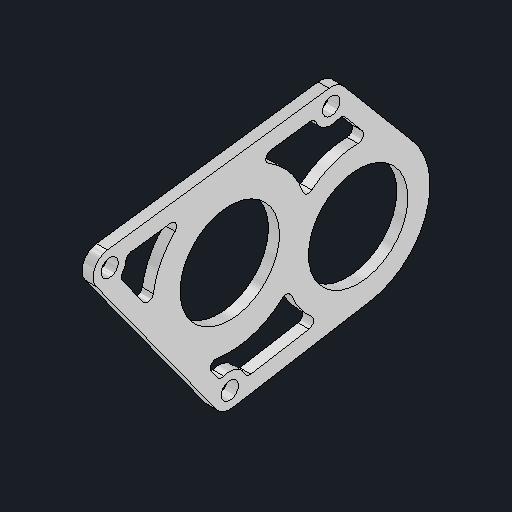
# Autodesk Inventor part: PLATE,BEARING,MOUNT
Saved by Autodesk Inventor 2026.1 (Build 301233020, 233B)
## iProperties
Created: 2026-01-27
Part Number: PLATE,BEARING,MOUNT
Material: Aluminum 3003-H16
Document SubType Name: Sheet Metal
Designer: Owen L
Density: 2.73809 g/cm^3
Sheet Metal Rule: Default
Appearance: Aluminum - Polished
Mass: 20.6939 g
Surface Area: 69.1803 cm^2
Volume: 7.55778 cm^3
Author: Owen L
Autodesk Inventor part; units mm, degrees
ref_plane "YZ Plane" through (0, 0, 0) normal (1, 0, 0) x (0, 1, 0)
ref_plane "XZ Plane" through (0, 0, 0) normal (0, 1, 0) x (-1, 0, 0)
ref_plane "XY Plane" through (0, 0, 0) normal (0, 0, 1) x (1, 0, 0)
sketch "Sketch1" plane through (0, 0, 0) normal (1, 0, 0) x (0, 1, 0)
  line L0 (0, -278.2902) -> (0, 46.3817) construction
  line L1 (36.388, -206.3665) -> (0, 0) construction
  arc A0 (16.0424, -209.8254) -> (49.6755, -222.1573) centre (36.388, -206.3665) ccw
  line L2 (61.8586, -134.906) -> (45.7568, -169.4363) construction
  arc A1 (66.5803, -134.2844) -> (59.0717, -131.044) centre (61.8586, -134.906) ccw
  arc A2 (73.3134, -202.2667) -> (74.9688, -198.001) centre (70.247, -198.6226) ccw
  arc A3 (11.22, -165.5743) -> (9.3117, -170.2345) centre (14.0068, -169.4363) ccw
  line L3 (66.5803, -134.2844) -> (74.9688, -198.001)
  line L4 (73.3134, -202.2667) -> (49.6755, -222.1573)
  line L5 (16.0424, -209.8254) -> (9.3117, -170.2345)
  line L6 (70.247, -198.6226) -> (45.7568, -169.4363) construction
  line L7 (59.0717, -131.044) -> (11.22, -165.5743)
  line L8 (45.7568, -169.4363) -> (14.0068, -169.4363) construction
  dimension "d8" = 209.55
  dimension "d9" = 175.506
  dimension "d11" = 10
  dimension "d12" = 20.6375
  dimension "d13" = 38.1
  dimension "d14" = 25
  dimension "d19" = 4.7625
  dimension "d37" = 40
  dimension "d39" = 90
  dimension "d40" = 31.75
  dimension "d41" = 38.1
  constraints: 16 end point, 8 point on circle, 8 tangent, 5 coincident, 4 centre point, 2 equal radius, 1 equal length
  measures "d8" distance of L1.end L1.start
  measures "d9" distance of L1.end L2.end
  measures "d11" angle of L0 L1
  measures "d12" radius of A0
  measures "d13" distance of L2.end L2.start
  measures "d14" angle of L0 L2
  measures "d19" radius of A1
  measures "d37" angle of L0 L6
  measures "d39" angle of L0 L8
  measures "d40" distance of L8.start L8.end
  measures "d41" distance of L1.start L2.end
extrude "Plate1" add sketch "Sketch1" along normal blind 3.175
hole "Hole1" at (0, 61.8586, -134.906) at (0, 14.0068, -169.4363) at (0, 70.247, -198.6226) direction (1, 0, 0) diameter 4.9784 end through all clearance for "Flat Head Machine Screw (82)" size "#10" standard "Ansi Unified Screw Threads"
hole "Hole2" at (0, 36.388, -206.3665) at (0, 45.7568, -169.4363) direction (1, 0, 0) diameter 28.575 end through all
sketch "Sketch2" plane through (3.175, 0, 0) normal (1, 0, 0) x (0, 0, -1)
  circle A0 centre (169.4363, 45.7568) radius 14.2875 projected
  circle A1 centre (206.3665, 36.388) radius 14.2875 projected
  circle A2 centre (198.6226, 70.247) radius 2.4892 projected
  circle A3 centre (169.4363, 14.0068) radius 2.4892 projected
  circle A4 centre (134.906, 61.8586) radius 2.4892 projected
  arc A5 (134.2844, 66.5803) -> (131.044, 59.0717) centre (134.906, 61.8586) ccw projected
  line L0 (165.5743, 11.22) -> (131.044, 59.0717) projected
  arc A6 (165.5743, 11.22) -> (170.2345, 9.3117) centre (169.4363, 14.0068) ccw projected
  line L1 (209.8254, 16.0424) -> (170.2345, 9.3117) projected
  arc A7 (209.8254, 16.0424) -> (222.1573, 49.6755) centre (206.3665, 36.388) ccw projected
  line L2 (202.2667, 73.3134) -> (222.1573, 49.6755) projected
  arc A8 (202.2667, 73.3134) -> (198.001, 74.9688) centre (198.6226, 70.247) ccw projected
  line L3 (134.2844, 66.5803) -> (198.001, 74.9688) projected
  line L4 (134.906, 61.8586) -> (198.6226, 70.247)
  line L5 (198.6226, 70.247) -> (218.5132, 46.6091)
  arc A9 (209.0271, 20.7375) -> (218.5132, 46.6091) centre (206.3665, 36.388) ccw
  line L6 (209.0271, 20.7375) -> (169.4363, 14.0068)
  line L7 (169.4363, 14.0068) -> (134.906, 61.8586)
  circle A10 centre (134.906, 61.8586) radius 4.7625
  circle A11 centre (198.6226, 70.247) radius 4.7625
  circle A12 centre (169.4363, 14.0068) radius 4.7625
  circle A13 centre (169.4363, 45.7568) radius 22.225
  circle A14 centre (206.3665, 36.388) radius 20.6375
  point P0 (0, 0)
  point P1 (196.0269, 18.5274)
  point P2 (186.3547, 31.3444)
  point P3 (161.5078, 24.9941)
  point P4 (166.6495, 17.8688)
  point P5 (174.1315, 14.805)
  point P6 (191.1791, 50.3612)
  point P7 (210.0229, 56.699)
  point P8 (201.689, 66.603)
  point P9 (193.9009, 69.6254)
  point P10 (175.3438, 67.1823)
  point P11 (147.233, 44.776)
  point P12 (158.1848, 64.9233)
  point P13 (139.6278, 62.4802)
  point P14 (137.6928, 57.9966)
  dimension "d42" = 4.7625
  dimension "d44" = 41.275
  dimension "d45" = 44.45
  constraints: 8 end point, 6 centre point, 5 coincident, 3 concentric, 2 point on circle, 4 other
  measures "d42" distance between parallel lines of L0 L7
  measures "d44" diameter of A14
  measures "d45" diameter of A13
extrude "Cut1" cut sketch "Sketch2" against normal blind 3.175 contours A11 L5 A14 A13 L4 | A13 L7 A10 L4 | A14 L6 A12 L7 A13
fillet "Corner Round1" radius 1.5875 14 edges at (1.5875, 44.776, -147.233) (1.5875, 64.9233, -158.1848) (1.5875, 57.9966, -137.6928) (1.5875, 56.699, -210.0229) (1.5875, 31.3444, -186.3547) (1.5875, 14.805, -174.1315) (1.5875, 18.5274, -196.0269) (1.5875, 50.3612, -191.1791) (1.5875, 62.4802, -139.6278) (1.5875, 69.6254, -193.9009) (1.5875, 66.603, -201.689) (1.5875, 67.1823, -175.3438) (1.5875, 17.8688, -166.6495) (1.5875, 24.9941, -161.5078)
equation "\"d25\" = Thickness"
equation "\"d46\" = Thickness"
equation "\"d7\" = Thickness"
equation "\"BendRadius\" = Thickness"
equation "\"BendReliefWidth\" = Thickness"
equation "\"BendReliefDepth\" = 0.5 * Thickness"
equation "\"CornerReliefSize\" = 4 * Thickness"
equation "\"MinimumRemnant\" = 2 * Thickness"
equation "\"TransitionRadius\" = BendRadius"
equation "\"JacobiRadiusSize\" = BendRadius"
equation "\"GapSize\" = Thickness"
equation "\"Thickness\" = 3.175"
body "Solid1"
